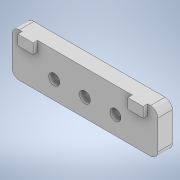
# Autodesk Inventor part: charger_holder
Saved by Autodesk Inventor 2022.1 (Build 261234000, 234)
## iProperties
Created: 2021-07-19
Part Number: charger_holder
Material: Generic
Document SubType Name: Modeling
Designer: dwbertol
Density: 1 g/cm^3
Appearance: Default
Author: dwbertol
## iProperties of the stored document charger_holder_3DPrint.ipt
Created: 2021-07-19
Part Number: charger_holder_3DPrint
Material: Generic
Document SubType Name: Modeling
Designer: dwbertol
Density: 1 g/cm^3
Appearance: Default
Author: dwbertol
Autodesk Inventor part; units mm, degrees
ref_plane "YZ Plane" through (0, 0, 0) normal (1, 0, 0) x (0, 1, 0)
ref_plane "XZ Plane" through (0, 0, 0) normal (0, 1, 0) x (-1, 0, 0)
ref_plane "XY Plane" through (0, 0, 0) normal (0, 0, 1) x (1, 0, 0)
sketch "Sketch1" plane through (0, 0, 0) normal (0, 0, 1) x (1, 0, 0)
  line L0 (-10, 3) -> (10, 3)
  line L1 (10, 3) -> (10, -3)
  line L2 (10, -3) -> (-10, -3)
  line L3 (-10, -3) -> (-10, 3)
  circle A0 centre (-4.2, -0.5) radius 0.75
  circle A1 centre (4.2, -0.5) radius 0.75
  circle A2 centre (0, -0.5) radius 0.75
  point P0 (0, 0)
  dimension "d0" = 20
  dimension "d1" = 6
  dimension "d2" = 3
  dimension "d3" = 10
  dimension "d7" = 1.5
  dimension "d8" = 1.5
  dimension "d18" = 2.5
  dimension "d19" = 2.5
  dimension "d20" = 1.5
  dimension "d21" = 2.5
  dimension "d22" = 10
  dimension "d23" = 4.2
  dimension "d24" = 4.2
  constraints: 8 end point, 3 centre point, 2 parallel, 1 horizontal, 1 perpendicular
  measures "d0" distance between parallel lines of L1 L3
  measures "d1" distance between parallel lines of L2 L0
  measures "d2" distance from line of L0 point (0, 0)
  measures "d3" distance from line of point (0, 0) L3
  measures "d7" diameter of A0
  measures "d8" diameter of A1
  measures "d18" distance from line of A1.centre L2
  measures "d19" distance from line of A0.centre L2
  measures "d20" diameter of A2
  measures "d21" distance from line of L2 A2.centre
  measures "d22" distance from line of L3 A2.centre
  measures "d23" distance of A2.centre A0.centre
  measures "d24" distance of A1.centre A2.centre
extrude "Extrusion1" add sketch "Sketch1" along normal mid plane 2
sketch "Sketch2" plane through (0, 0, 1) normal (0, 0, 1) x (1, 0, 0)
  line L0 (10, 3) -> (-10, 3) projected
  line L1 (-8.6, 3) -> (-6.5, 3)
  line L2 (-6.5, 3) -> (-6.5, 1.6)
  line L3 (-6.5, 1.6) -> (-8.6, 1.6)
  line L4 (-8.6, 1.6) -> (-8.6, 3)
  line L5 (6.5, 3) -> (8.6, 3)
  line L6 (8.6, 3) -> (8.6, 1.6)
  line L7 (8.6, 1.6) -> (6.5, 1.6)
  line L8 (6.5, 1.6) -> (6.5, 3)
  line L9 (-10, 3) -> (-10, -3) projected
  line L10 (10, -3) -> (10, 3) projected
  point P0 (0, 0)
  point P1 (-6.5, 2.3)
  dimension "d17" = 1.4
  dimension "d30" = 2.1
  dimension "d31" = 6.5
  dimension "d32" = 6.5
  dimension "d33" = 2.1
  constraints: 16 end point, 4 parallel, 3 point on line, 2 horizontal, 2 perpendicular, 1 midpoint
  measures "d17" distance between parallel lines of L0 L3
  measures "d30" distance between parallel lines of L2 L4
  measures "d31" horizontal distance of point (0, 0) point (-6.5, 2.3)
  measures "d32" distance from line of L8 point (0, 0)
  measures "d33" distance from line of L8 L6.end
extrude "Extrusion2" add sketch "Sketch2" along normal blind 0.6
fillet "Fillet1" radius 1 4 edges at (10, 3, 0) (10, -3, 0) (-10, -3, 0) (-10, 3, 0)
equation "\"d2\" = 0.5 * d1"
equation "\"d3\" = 0.5 * d0"
equation "\"d7\" = d20"
equation "\"d8\" = d20"
equation "\"d19\" = d18"
equation "\"d21\" = d19"
equation "\"d22\" = d3"
equation "\"d24\" = d23"
equation "\"d32\" = d31"
equation "\"d33\" = d30"
body "Solid1"
